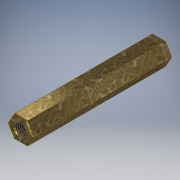
# Autodesk Inventor part: Part3_Poste largo de latón
Saved by Autodesk Inventor 2019 (Build 230136000, 136)
## iProperties
Created: 2023-05-02
Part Number: Part3_Poste largo de latón
Material: Generic
Document SubType Name: Modeling
Designer: Tecneu Technology
Density: 1 g/cm^3
Appearance: Foil Gold
Author: Tecneu Technology
Autodesk Inventor part; units mm, degrees
ref_plane "YZ Plane" through (0, 0, 0) normal (1, 0, 0) x (0, 1, 0)
ref_plane "XZ Plane" through (0, 0, 0) normal (0, 1, 0) x (-1, 0, 0)
ref_plane "XY Plane" through (0, 0, 0) normal (0, 0, 1) x (1, 0, 0)
sketch "Sketch1" plane through (0, 0, 0) normal (0, 0, 1) x (1, 0, 0)
  line L0 (1.3712, 2.375) -> (2.7424, 0)
  line L1 (2.7424, 0) -> (1.3712, -2.375)
  line L2 (1.3712, -2.375) -> (-1.3712, -2.375)
  line L3 (-1.3712, -2.375) -> (-2.7424, 0)
  line L4 (-2.7424, 0) -> (-1.3712, 2.375)
  line L5 (-1.3712, 2.375) -> (1.3712, 2.375)
  circle A0 centre (0, 0) radius 1.175
  dimension "d0" = 4.75
  dimension "d1" = 2.35
  constraints: 12 end point, 2 coincident, 1 centre point, 13 other
  measures "d0" distance between parallel lines of L2 L5
  measures "d1" diameter of A0
extrude "Extrusion1" add sketch "Sketch1" along normal blind 30
thread "Thread1" size "M2.5x0.45" class "6H" standard "ANSI Metric M Profile" full length
chamfer "Chamfer1" distance 0.25 angle 45 14 edges at (0, 2.375, 30) (-2.0568, 1.1875, 30) (-2.0568, -1.1875, 30) (2.0568, -1.1875, 30) (2.0568, 1.1875, 30) (2.0568, 1.1875, 0) (0, 2.375, 0) (-2.0568, 1.1875, 0) (-2.0568, -1.1875, 0) (-1.175, 0, 0) (0, -2.375, 0) (2.0568, -1.1875, 0) (-1.175, 0, 30) (0, -2.375, 30)
body "Solid1"
